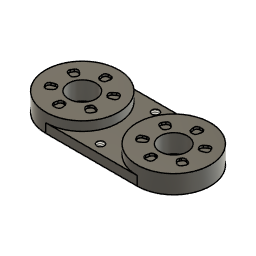
Challenge Exercise 3 model v1 (Autodesk Fusion 360 design; units mm, degrees)
Autodesk Fusion 360 part; units mm, degrees
note: some values were not read from the file. Set by a fixed rule: which sketch regions a step uses.
sketch "Sketch1" plane through (0, 0, 0) normal (0, 1, 0) x (1, 0, 0)
  circle A0 centre (-31.75, 0) radius 25.4
  circle A1 centre (31.75, 0) radius 25.4
  line L0 (-31.75, 0) -> (31.75, 0) construction
  line L1 (-31.75, 25.4) -> (31.75, 25.4)
  line L2 (-31.75, -25.4) -> (31.75, -25.4)
  dimension "d1" = 63.5
  dimension "d2" = 50.8
  constraint coincident A1.centre L0.end
  constraint midpoint origin L0
  constraint equal A0 A1
  constraint coincident A0.centre L0.start
  constraint horizontal L0
  constraint coincident A0 L1.start
  constraint coincident A1 L1.end
  constraint tangent A1 L1
  constraint coincident A0 L2.start
  constraint coincident A1 L2.end
  constraint tangent A1 L2
  constraint tangent A0 L1
  constraint tangent A0 L2
  measures "d1" distance of A0.centre A1.centre
  measures "d2" diameter of A0
extrude "Extrude1" add sketch "Sketch1" along normal blind 6.35
extrude "Extrude2" add sketch "Sketch1" along normal blind 12.7 contours A0 | A1
sketch "Sketch2" plane through (0, 12.7, 0) normal (0, 1, 0) x (-1, 0, 0)
  circle A0 centre (31.75, 0) radius 25.4
  line L0 (31.75, 0) -> (31.75, -19.05) construction
  circle A1 centre (31.75, 0) radius 19.05
  circle A2 centre (31.75, 0) radius 12.7
  line L1 (29.5447, -12.5071) -> (28.442, -18.7606)
  line L2 (33.9553, -12.5071) -> (35.058, -18.7606)
  dimension "d7" = 25.4
  dimension "d8" = 38.1
  dimension "d9" = 10
  dimension "d10" = 10
  constraint coincident A0.centre L0.start
  constraint vertical L0
  constraint coincident L0.end A1
  constraint coincident A2 L1.start
  constraint coincident A1 L1.end
  constraint coincident A2 L2.start
  constraint coincident A1 L2.end
  constraint coincident A0.centre L2
  constraint coincident A0.centre L1
  measures "d7" diameter of A2
  measures "d8" diameter of A1
  measures "d9" angle of L0 L2
  measures "d10" angle of L0 L1
extrude "Extrude3" cut sketch "Sketch2" against normal blind 1.5875 contours A1 A2 L1 L2 picked at (33.468, -16.819)
fillet "Fillet1" radius 2.032 4 edges at (-29.5447, 11.9062, -12.5071) (-33.9553, 11.9062, -12.5071) (-35.058, 11.9062, -18.7606) (-28.442, 11.9062, -18.7606)
pattern_circular "C-Pattern1" count 6 over 360 about axis through (-31.75, 12.7, 0) along (0, 1, 0) of "Extrude3", "Fillet1"
mirror "Mirror1" about plane through (0, 0, 0) normal (1, 0, 0) of "Extrude3", "Fillet1", "C-Pattern1"
sketch "Sketch3" plane through (0, 12.7, 0) normal (0, 1, 0) x (-1, 0, 0)
  arc A0 (20.5291, -5.9482) -> (20.9882, -6.7435) centre (31.75, 0) ccw
  arc A1 (20.5725, -9.379) -> (20.9882, -6.7435) centre (19.2664, -7.8224) ccw
  line L0 (20.5725, -9.379) -> (18.8067, -10.8607)
  arc A2 (15.7992, -10.415) -> (18.8067, -10.8607) centre (17.5006, -9.3041) ccw
  arc A3 (14.7549, -8.6063) -> (15.7992, -10.415) centre (31.75, 0) ccw
  arc A4 (15.8727, -5.7789) -> (14.7549, -8.6063) centre (16.5677, -7.6883) ccw
  line L1 (15.8727, -5.7789) -> (18.0388, -4.9905)
  arc A5 (20.5291, -5.9482) -> (18.0388, -4.9905) centre (18.7338, -6.8999) ccw
  arc A6 (20.9882, 6.7435) -> (20.5291, 5.9482) centre (31.75, 0) ccw
  arc A7 (18.0388, 4.9905) -> (20.5291, 5.9482) centre (18.7338, 6.8999) ccw
  line L2 (18.0388, 4.9905) -> (15.8727, 5.7789)
  arc A8 (14.7549, 8.6063) -> (15.8727, 5.7789) centre (16.5677, 7.6883) ccw
  arc A9 (15.7992, 10.415) -> (14.7549, 8.6063) centre (31.75, 0) ccw
  arc A10 (18.8067, 10.8607) -> (15.7992, 10.415) centre (17.5006, 9.3041) ccw
  line L3 (18.8067, 10.8607) -> (20.5725, 9.379)
  arc A11 (20.9882, 6.7435) -> (20.5725, 9.379) centre (19.2664, 7.8224) ccw
  arc A12 (32.2091, 12.6917) -> (31.2909, 12.6917) centre (31.75, 0) ccw
  arc A13 (29.2163, 14.3695) -> (31.2909, 12.6917) centre (31.2174, 14.7224) ccw
  line L4 (29.2163, 14.3695) -> (28.816, 16.6396)
  arc A14 (30.7057, 19.0214) -> (28.816, 16.6396) centre (30.8171, 16.9924) ccw
  arc A15 (32.7943, 19.0214) -> (30.7057, 19.0214) centre (31.75, 0) ccw
  arc A16 (34.684, 16.6396) -> (32.7943, 19.0214) centre (32.6829, 16.9924) ccw
  line L5 (34.684, 16.6396) -> (34.2837, 14.3695)
  arc A17 (32.2091, 12.6917) -> (34.2837, 14.3695) centre (32.2826, 14.7224) ccw
  arc A18 (42.9709, 5.9482) -> (42.5118, 6.7435) centre (31.75, 0) ccw
  arc A19 (42.9275, 9.379) -> (42.5118, 6.7435) centre (44.2336, 7.8224) ccw
  line L6 (42.9275, 9.379) -> (44.6933, 10.8607)
  arc A20 (47.7008, 10.415) -> (44.6933, 10.8607) centre (45.9994, 9.3041) ccw
  arc A21 (48.7451, 8.6063) -> (47.7008, 10.415) centre (31.75, 0) ccw
  arc A22 (47.6273, 5.7789) -> (48.7451, 8.6063) centre (46.9323, 7.6883) ccw
  line L7 (47.6273, 5.7789) -> (45.4612, 4.9905)
  arc A23 (42.9709, 5.9482) -> (45.4612, 4.9905) centre (44.7662, 6.8999) ccw
  arc A24 (42.5118, -6.7435) -> (42.9709, -5.9482) centre (31.75, 0) ccw
  arc A25 (45.4612, -4.9905) -> (42.9709, -5.9482) centre (44.7662, -6.8999) ccw
  line L8 (45.4612, -4.9905) -> (47.6273, -5.7789)
  arc A26 (48.7451, -8.6063) -> (47.6273, -5.7789) centre (46.9323, -7.6883) ccw
  arc A27 (47.7008, -10.415) -> (48.7451, -8.6063) centre (31.75, 0) ccw
  arc A28 (44.6933, -10.8607) -> (47.7008, -10.415) centre (45.9994, -9.3041) ccw
  line L9 (44.6933, -10.8607) -> (42.9275, -9.379)
  arc A29 (42.5118, -6.7435) -> (42.9275, -9.379) centre (44.2336, -7.8224) ccw
  arc A30 (31.2909, -12.6917) -> (32.2091, -12.6917) centre (31.75, 0) ccw
  arc A31 (34.2837, -14.3695) -> (32.2091, -12.6917) centre (32.2826, -14.7224) ccw
  line L10 (34.2837, -14.3695) -> (34.684, -16.6396)
  arc A32 (32.7943, -19.0214) -> (34.684, -16.6396) centre (32.6829, -16.9924) ccw
  arc A33 (30.7057, -19.0214) -> (32.7943, -19.0214) centre (31.75, 0) ccw
  arc A34 (28.816, -16.6396) -> (30.7057, -19.0214) centre (30.8171, -16.9924) ccw
  line L11 (28.816, -16.6396) -> (29.2163, -14.3695)
  arc A35 (31.2909, -12.6917) -> (29.2163, -14.3695) centre (31.2174, -14.7224) ccw
  circle A36 centre (31.75, 0) radius 25.4
  circle A37 centre (31.75, 0) radius 9.525
  dimension "d17" = 19.05
  constraint concentric A0 A37
  measures "d17" diameter of A37
extrude "Extrude4" cut sketch "Sketch3" against normal through all contours A37
mirror "Mirror2" about plane through (0, 0, 0) normal (1, 0, 0) of "Extrude4"
sketch "Sketch4" plane through (0, 6.35, 0) normal (0, 1, 0) x (-1, 0, 0)
  arc A0 (-31.75, -25.4) -> (-31.75, 25.4) centre (-31.75, 0) ccw
  line L0 (-31.75, -25.4) -> (31.75, -25.4)
  arc A1 (31.75, 25.4) -> (31.75, -25.4) centre (31.75, 0) ccw
  line L1 (31.75, 25.4) -> (-31.75, 25.4)
  point P0 (0, -19.05)
  point P1 (0, 19.05)
  dimension "d20" = 19.05
  dimension "d21" = 19.05
  constraint vertical origin P0
  constraint vertical origin P1
  measures "d20" distance of origin P1
  measures "d21" distance of origin P0
hole "Hole1" at (0, 6.35, -19.05) at (0, 6.35, 19.05) direction (0, -1, 0) diameter 5.1308 depth 17.78 tip angle 118
thread "Thread1" "ANSI Unified Screw Threads 0.25 1/4-20 UNC 1B" thread offset 0 thread depth 10.0076
